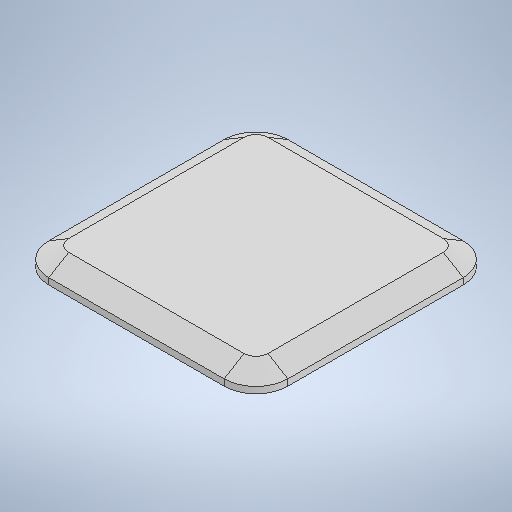
# Autodesk Inventor part: IMU_Base_T-Shirt
Saved by Autodesk Inventor 2025.2 (Build 292293000, 293)
## iProperties
Created: 2024-11-14
Part Number: IMU_Base_T-Shirt
Material: Generic
Document SubType Name: Modeling
Designer: matss
Density: 1 g/cm^3
Appearance: Default
Author: matss
Autodesk Inventor part; units mm, degrees
ref_plane "YZ Plane" through (0, 0, 0) normal (1, 0, 0) x (0, 1, 0)
ref_plane "XZ Plane" through (0, 0, 0) normal (0, 1, 0) x (-1, 0, 0)
ref_plane "XY Plane" through (0, 0, 0) normal (0, 0, 1) x (1, 0, 0)
sketch "Sketch1" plane through (0, 0, 0) normal (0, 1, 0) x (-1, 0, 0)
  line L0 (30, 30) -> (-30, 30)
  line L1 (-30, 30) -> (-30, -30)
  line L2 (-30, -30) -> (30, -30)
  line L3 (30, -30) -> (30, 30)
  point P0 (0, 0)
  point P1 (30, 0)
  point P2 (0, 30)
  dimension "d0" = 60
  dimension "d1" = 60
  constraints: 8 end point, 2 midpoint, 2 parallel, 1 horizontal, 1 horizontal alignment, 1 perpendicular, 1 vertical alignment
  measures "d0" distance of L2.end L0.start
  measures "d1" distance of L0.start L0.end
extrude "Extrusion1" add sketch "Sketch1" along normal blind 2
sketch "Sketch2" plane through (0, 2, 0) normal (0, 1, 0) x (1, 0, 0)
  line L0 (30, -30) -> (30, 30) projected
  line L1 (30, 30) -> (-30, 30) projected
  line L2 (-30, 30) -> (-30, -30) projected
  line L3 (-30, -30) -> (30, -30) projected
  line L4 (-30, 0) -> (30, 0)
  line L5 (0, -30) -> (0, 30)
  circle A0 centre (-12.5, -12.5) radius 4.25
  circle A1 centre (-12.5, 12.5) radius 4.25
  circle A2 centre (12.5, 12.5) radius 4.25
  circle A3 centre (12.5, -12.5) radius 4.25
  point P0 (0, 0)
  dimension "d13" = 8.5
  dimension "d14" = 25
  dimension "d15" = 25
  constraints: 4 centre point, 4 end point, 4 midpoint, 3 equal radius, 3 other
  measures "d13" diameter of A0
  measures "d14" distance of A3.centre A0.centre
  measures "d15" distance of A1.centre A0.centre
extrude "Extrusion2" add sketch "Sketch2" along normal blind 2
sketch "Sketch3" plane through (0, 4, 0) normal (0, 1, 0) x (1, 0, 0)
  line L0 (-30, 30) -> (-30, -30) projected
  line L1 (-30, -30) -> (30, -30) projected
  line L2 (30, -30) -> (30, 30) projected
  line L3 (30, 30) -> (-30, 30) projected
  point P0 (0, 0)
extrude "Extrusion3" add sketch "Sketch3" along normal blind 0.6
fillet "Fillet1" radius 8 4 edges at (30, 2.3, 30) (-30, 2.3, 30) (-30, 2.3, -30) (30, 2.3, -30)
chamfer "Chamfer1" distance 5 distance2 3 8 edges at (0, 4.6, 30) (27.6569, 4.6, 27.6569) (30, 4.6, 0) (27.6569, 4.6, -27.6569) (0, 4.6, -30) (-27.6569, 4.6, -27.6569) (-30, 4.6, 0) (-27.6569, 4.6, 27.6569) measured on face at (27.3033, 4.6, -27.3033) measured on face at (0, 4.6, 29.5) measured on face at (-29.5, 4.6, 0) measured on face at (0, 4.6, -29.5) measured on face at (29.5, 4.6, 0) measured on face at (-27.3033, 4.6, -27.3033) measured on face at (27.3033, 4.6, 27.3033) measured on face at (-27.3033, 4.6, 27.3033)
sketch "Sketch4" plane through (0, 0, 0) normal (0, -1, 0) x (1, 0, 0)
  arc A0 (25, 22) -> (22, 25) centre (22, 22) ccw construction
  arc A1 (-25, -22) -> (-22, -25) centre (-22, -22) ccw construction
  line L0 (22, 22) -> (-22, -22) construction
  arc A2 (-22, 25) -> (-25, 22) centre (-22, 22) ccw construction
  arc A3 (22, -25) -> (25, -22) centre (22, -22) ccw construction
  line L1 (-22, 22) -> (22, -22) construction
  point P0 (0, 0)
  point P1 (0, 0)
  constraints: 4 end point, 1 coincident
body "Solid1"
